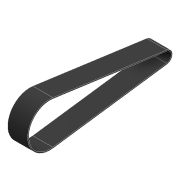
# Autodesk Inventor part: Ременная передача
Saved by Autodesk Inventor 2022 (Build 260153000, 153)
## iProperties
Created: 2023-02-20
Part Number: Ременная передача
Material: Типовые
Document SubType Name: Modeling
Designer: Глеб
Density: 1 g/cm^3
Appearance: Резина — черная
Author: Глеб
Autodesk Inventor part; units mm, degrees
ref_plane "YZ Plane" through (0, 0, 0) normal (1, 0, 0) x (0, 1, 0)
ref_plane "XZ Plane" through (0, 0, 0) normal (0, 1, 0) x (-1, 0, 0)
ref_plane "XY Plane" through (0, 0, 0) normal (0, 0, 1) x (1, 0, 0)
sketch "Эскиз1" plane through (0, 0, 0) normal (1, 0, 0) x (0, 1, 0)
  circle A0 centre (0, 0) radius 10.5
  line L0 (0, -71.7) -> (0, 24.2) construction
  circle A1 centre (0, -55) radius 3
  line L1 (2.972, -55.4091) -> (10.4019, -1.4318)
  line L2 (-10.4019, -1.4318) -> (-2.972, -55.4091)
  circle A2 centre (0, 0) radius 10
  circle A3 centre (0, -55) radius 2.5
  line L3 (9.9066, -1.3636) -> (2.4766, -55.3409)
  line L4 (-2.4766, -55.3409) -> (-9.9066, -1.3636)
  dimension "d0" = 21
  dimension "d1" = 6
  dimension "d2" = 55
  dimension "d3" = 20
  dimension "d4" = 5
  constraints: 8 end point, 8 point on circle, 8 tangent, 4 centre point, 3 coincident, 1 point on line
  measures "d0" diameter of A0
  measures "d1" diameter of A1
  measures "d2" distance of A0.centre A1.centre
  measures "d3" diameter of A2
  measures "d4" diameter of A3
extrude "Выдавливание1" add sketch "Эскиз1" along normal mid plane 9.5 contours A0 L3 A2 L4 | A0 L4 A1 L2 | L1 A1 L3 A0 | A1 L4 A3 L3 picked at (10.1468, 1.5856) picked at (-2.6945, -54.4287)
